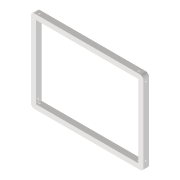
# Autodesk Inventor part: Omniscope_USBC_Wellplatemount
Saved by Autodesk Inventor 2022 (Build 260153000, 153)
## iProperties
Created: 2023-05-17
Part Number: Omniscope_USBC_Wellplatemount
Material: Generisch
Document SubType Name: Modeling
Designer: diederichbenedict
Density: 1 g/cm^3
Appearance: Vorgabe
Author: diederichbenedict
Autodesk Inventor part; units mm, degrees
ref_plane "YZ Plane" through (0, 0, 0) normal (1, 0, 0) x (0, 1, 0)
ref_plane "XZ Plane" through (0, 0, 0) normal (0, 1, 0) x (-1, 0, 0)
ref_plane "XY Plane" through (0, 0, 0) normal (0, 0, 1) x (1, 0, 0)
sketch "Skizze1" plane through (0, 0, 0) normal (0, 0, 1) x (1, 0, 0)
  line L0 (-61.9244, 60.0948) -> (74.9176, 60.0948) construction
  arc A0 (85.9176, 49.0948) -> (74.9176, 60.0948) centre (74.9176, 49.0948) ccw construction
  line L1 (85.9176, 49.0948) -> (85.9176, 38.1005) construction
  line L2 (85.9176, 38.1005) -> (78.8171, 31) construction
  line L3 (78.8171, -29.3201) -> (85.9176, -36.4206) construction
  line L4 (85.9176, -36.4206) -> (85.9176, -44.1557) construction
  arc A1 (74.9176, -55.1557) -> (85.9176, -44.1557) centre (74.9176, -44.1557) ccw construction
  arc A2 (-72.9244, -44.1557) -> (-61.9244, -55.1557) centre (-61.9244, -44.1557) ccw construction
  line L5 (-72.9244, -44.1557) -> (-72.9244, -36.4206) construction
  line L6 (-65.8239, 31) -> (-72.9244, 38.1005) construction
  line L7 (-72.9244, 38.1005) -> (-72.9244, 49.0948) construction
  arc A3 (-61.9244, 60.0948) -> (-72.9244, 49.0948) centre (-61.9244, 49.0948) ccw construction
  line L8 (-67.9244, 60.0948) -> (80.9176, 60.0948)
  line L9 (85.9176, 55.0948) -> (85.9176, -51.7356)
  line L10 (80.9176, -56.7356) -> (-67.9244, -56.7356)
  line L11 (-72.9244, -51.7356) -> (-72.9244, 55.0948)
  arc A4 (-67.9244, 60.0948) -> (-72.9244, 55.0948) centre (-67.9244, 55.0948) ccw
  arc A5 (85.9176, 55.0948) -> (80.9176, 60.0948) centre (80.9176, 55.0948) ccw
  arc A6 (80.9176, -56.7356) -> (85.9176, -51.7356) centre (80.9176, -51.7356) ccw
  arc A7 (-72.9244, -51.7356) -> (-67.9244, -56.7356) centre (-67.9244, -51.7356) ccw
  line L12 (-65.9244, -49.7356) -> (78.9176, -49.7356)
  line L13 (78.9176, -49.7356) -> (78.9176, 53.0948)
  line L14 (78.9176, 53.0948) -> (-65.9244, 53.0948)
  line L15 (-65.9244, 53.0948) -> (-65.9244, -49.7356)
  dimension "d3" = 5
  dimension "d42" = 158.842
  dimension "d43" = 116.8304
  dimension "d45" = 7
  dimension "d46" = 7
  dimension "d47" = 7
  dimension "d48" = 7
  constraints: 32 end point, 16 point on circle, 8 centre point, 8 tangent, 4 parallel, 3 equal radius, 2 horizontal, 2 perpendicular
  measures "d3" radius of A4
  measures "d42" distance between parallel lines of L9 L11
  measures "d43" distance between parallel lines of L0 L10
  measures "d45" distance between parallel lines of L10 L12
  measures "d46" distance between parallel lines of L8 L14
  measures "d47" distance between parallel lines of L7 L15
  measures "d48" distance between parallel lines of L9 L13
extrude "Extrusion1" add sketch "Skizze1" along normal blind 8
sketch "Skizze4" plane through (-67.9244, 60.0948, 8) normal (0, 1, 0) x (1, 0, 0)
  circle A0 centre (143.842, -102.2347) radius 1.4 projected
  circle A1 centre (5, -102.2347) radius 1.4 projected
  line L0 (148.842, -98.2347) -> (0, -98.2347) projected
  line L1 (0, -98.2347) -> (0, -106.2347) projected
  line L2 (148.842, -106.2347) -> (0, -106.2347) projected
  line L3 (148.842, -98.2347) -> (148.842, -106.2347) projected
  circle A2 centre (3.6, 3) radius 1.4
  circle A3 centre (143.842, 3) radius 1.4
  line L4 (148.842, 8) -> (0, 8) projected
  point P0 (67.9244, 8)
  dimension "d28" = 2.8
  dimension "d30" = 2.8
  dimension "d49" = 5
  constraints: 2 centre point
  measures "d28" diameter of A2
  measures "d30" diameter of A3
  measures "d49" distance from line of A2.centre L4
extrude "Extrusion3" cut sketch "Skizze4" against normal blind 20 contours A2 | A3
sketch "Skizze5" plane through (-67.9244, -56.7356, 8) normal (0, -1, 0) x (1, 0, 0)
  circle A0 centre (143.842, -3) radius 1.4 projected
  circle A1 centre (3.6, -3) radius 1.4 projected
  point P0 (67.9244, -8)
extrude "Extrusion4" cut sketch "Skizze5" against normal blind 20
sketch "Skizze6" plane through (85.9176, -51.7356, 8) normal (1, 0, 0) x (0, 0, -1)
  circle A0 centre (-102.2347, 101.8304) radius 1.4 projected
  circle A1 centre (-102.2347, 5) radius 1.4 projected
  circle A2 centre (3, 103.2304) radius 1.4
  circle A3 centre (3, 6.4) radius 1.4
  line L0 (14.9128, 45.7425) -> (14.9128, 109.8425)
  point P0 (8, 51.7356)
  point P1 (8, 111.8304)
  dimension "d35" = 2.8
  dimension "d37" = 2.8
  dimension "d50" = 5
  constraints: 2 centre point, 2 end point, 1 vertical, 2 other
  measures "d35" diameter of A2
  measures "d37" diameter of A3
  measures "d50" horizontal distance of A2.centre point (8, 111.83)
extrude "Extrusion5" cut sketch "Skizze6" against normal blind 20 contours A2 | A3
sketch "Skizze7" plane through (-72.9244, -51.7356, 8) normal (-1, 0, 0) x (0, 0, 1)
  line L0 (-4.4, -5) -> (-4.4, 2) projected
  circle A0 centre (-3, 6.4) radius 1.4 projected
  circle A1 centre (-3, 103.2304) radius 1.4 projected
  point P0 (-8, 51.7356)
extrude "Extrusion6" cut sketch "Skizze7" against normal blind 20
